Autodesk Inventor part; units mm, degrees
(part 3 of 3)
sketch "Эскиз17" plane through (0, 0, 0) normal (0, 0, -1) x (-1, 0, 0)
  arc A0 (-173.7802, -1.8121) -> (-173.9729, -1.8158) centre (-173.7802, -6.8121) ccw projected
  line L0 (-173.7802, -1.8121) -> (-160.0497, -1.8121) projected
  arc A1 (-152.9786, -18.8832) -> (-160.0497, -1.8121) centre (-160.0497, -11.8121) ccw projected
  line L1 (-152.9786, -18.8832) -> (-158.214, -24.1186) projected
  arc A2 (-164.3429, -27.0031) -> (-158.214, -24.1186) centre (-165.2851, -17.0475) ccw projected
  arc A3 (-173.9729, -1.8158) -> (-164.3429, -27.0031) centre (-132.2862, -0.3121) ccw projected
  line L2 (-174, 36.762) -> (-174, 1.1879) projected
  arc A4 (-171.0229, 35.5585) -> (-174, 36.762) centre (-174.2862, 31.7702) ccw projected
  arc A5 (-153.0118, 17.836) -> (-171.0229, 35.5585) centre (-295.6146, -109.0766) ccw projected
  arc A6 (-160.4818, 1.1879) -> (-153.0118, 17.836) centre (-160.4818, 11.1879) ccw projected
  line L3 (-160.4818, 1.1879) -> (-174, 1.1879) projected
  line L4 (-179, 51.6879) -> (181.2748, 51.6879) projected
  line L5 (-179, -0.3121) -> (-179, 51.6879) projected
  arc A7 (-179, -0.3121) -> (-165.3495, -33.3121) centre (-132.2862, -0.3121) ccw projected
  line L6 (-165.3495, -33.3121) -> (167.6243, -33.3121) projected
  arc A8 (167.6243, -33.3121) -> (181.2748, -0.3121) centre (134.5611, -0.3121) ccw projected
  line L7 (181.2748, 51.6879) -> (181.2748, -0.3121) projected
  line L8 (176.2748, 1.1879) -> (176.2748, 36.762) projected
  line L9 (176.2748, 1.1879) -> (162.7567, 1.1879) projected
  arc A9 (155.2866, 17.836) -> (162.7567, 1.1879) centre (162.7567, 11.1879) ccw projected
  arc A10 (173.2978, 35.5585) -> (155.2866, 17.836) centre (297.8894, -109.0766) ccw projected
  arc A11 (176.2748, 36.762) -> (173.2978, 35.5585) centre (176.5611, 31.7702) ccw projected
  arc A12 (-128.2552, 14.1361) -> (-136.3136, 14.1371) centre (-132.2862, -0.3121) ccw projected
  arc A13 (-145.382, 16.0725) -> (-136.3136, 14.1371) centre (-138.9985, 23.7699) ccw projected
  arc A14 (-168.1568, 38.4246) -> (-145.382, 16.0725) centre (-23.5217, 163.0162) ccw projected
  arc A15 (-164.3686, 46.6879) -> (-168.1568, 38.4246) centre (-164.3686, 41.6879) ccw projected
  line L10 (-164.3686, 46.6879) -> (-100.194, 46.6879) projected
  arc A16 (-96.4037, 38.427) -> (-100.194, 46.6879) centre (-100.194, 41.6879) ccw projected
  arc A17 (-119.19, 16.0661) -> (-96.4037, 38.427) centre (-240.0147, 161.9803) ccw projected
  arc A18 (-128.2552, 14.1361) -> (-119.19, 16.0661) centre (-125.5679, 23.7682) ccw projected
  arc A19 (170.4316, 38.4246) -> (166.6434, 46.6879) centre (166.6434, 41.6879) ccw projected
  arc A20 (147.6568, 16.0725) -> (170.4316, 38.4246) centre (25.7966, 163.0162) ccw projected
  arc A21 (138.5884, 14.1371) -> (147.6568, 16.0725) centre (141.2733, 23.7699) ccw projected
  arc A22 (138.5884, 14.1371) -> (130.53, 14.1361) centre (134.5611, -0.3121) ccw projected
  arc A23 (121.4649, 16.0661) -> (130.53, 14.1361) centre (127.8427, 23.7682) ccw projected
  arc A24 (98.6785, 38.427) -> (121.4649, 16.0661) centre (242.2895, 161.9803) ccw projected
  arc A25 (102.4688, 46.6879) -> (98.6785, 38.427) centre (102.4688, 41.6879) ccw projected
  line L11 (102.4688, 46.6879) -> (166.6434, 46.6879) projected
  arc A26 (77.8151, 38.3038) -> (74.1343, 46.6879) centre (74.1343, 41.6879) ccw projected
  line L12 (77.8151, 38.3038) -> (51.7107, 9.911) projected
  arc A27 (36.9877, 9.911) -> (51.7107, 9.911) centre (44.3492, 16.6792) ccw projected
  line L13 (36.9877, 9.911) -> (10.8834, 38.3038) projected
  arc A28 (14.5641, 46.6879) -> (10.8834, 38.3038) centre (14.5641, 41.6879) ccw projected
  line L14 (14.5641, 46.6879) -> (74.1343, 46.6879) projected
  line L15 (-49.4359, 9.911) -> (-75.5403, 38.3038) projected
  arc A29 (-71.8595, 46.6879) -> (-75.5403, 38.3038) centre (-71.8595, 41.6879) ccw projected
  line L16 (-71.8595, 46.6879) -> (-12.2893, 46.6879) projected
  arc A30 (-8.6085, 38.3038) -> (-12.2893, 46.6879) centre (-12.2893, 41.6879) ccw projected
  line L17 (-8.6085, 38.3038) -> (-34.7129, 9.911) projected
  arc A31 (-49.4359, 9.911) -> (-34.7129, 9.911) centre (-42.0744, 16.6792) ccw projected
  arc A32 (166.6178, -27.0031) -> (176.2477, -1.8158) centre (134.5611, -0.3121) ccw projected
  arc A33 (160.4889, -24.1186) -> (166.6178, -27.0031) centre (167.5599, -17.0475) ccw projected
  line L18 (160.4889, -24.1186) -> (155.2534, -18.8832) projected
  arc A34 (162.3245, -1.8121) -> (155.2534, -18.8832) centre (162.3245, -11.8121) ccw projected
  line L19 (162.3245, -1.8121) -> (176.055, -1.8121) projected
  arc A35 (176.2477, -1.8158) -> (176.055, -1.8121) centre (176.055, -6.8121) ccw projected
  circle A36 centre (-85.2862, 46.6879) radius 2.1 projected
  circle A37 centre (1.1374, 46.6879) radius 2.1 projected
  circle A38 centre (87.5611, 46.6879) radius 2.1 projected
  circle A39 centre (-123.2862, -0.3121) radius 2.1 projected
  circle A40 centre (-132.2862, 8.6879) radius 2.1 projected
  circle A41 centre (125.5611, -0.3121) radius 2.1 projected
  circle A42 centre (134.5611, -9.3121) radius 2.1 projected
  circle A43 centre (134.5611, 8.6879) radius 2.1 projected
  circle A44 centre (-132.2862, -0.3121) radius 4 projected
  circle A45 centre (-132.2862, -9.3121) radius 2.1 projected
  circle A46 centre (-141.2862, -0.3121) radius 2.1 projected
  circle A47 centre (143.5611, -0.3121) radius 2.1 projected
  circle A48 centre (134.5611, -0.3121) radius 4 projected
  line L20 (129.2891, -28.3121) -> (116.1593, -28.3121) projected
  arc A49 (114.1289, -23.1036) -> (116.1593, -28.3121) centre (116.1593, -25.3121) ccw projected
  arc A50 (116.4129, -21.0376) -> (114.1289, -23.1036) centre (243.3255, -163.6405) ccw projected
  arc A51 (131.9582, -23.9426) -> (116.4129, -21.0376) centre (123.0611, -28.5077) ccw projected
  arc A52 (129.2891, -28.3121) -> (131.9582, -23.9426) centre (129.2891, -25.3121) ccw projected
  line L21 (153.1971, -28.3121) -> (139.6296, -28.3121) projected
  arc A53 (136.8733, -24.1278) -> (139.6296, -28.3121) centre (139.6296, -25.3121) ccw projected
  arc A54 (153.1321, -21.0045) -> (136.8733, -24.1278) centre (146.0611, -28.0756) ccw projected
  line L22 (153.1321, -21.0045) -> (155.3184, -23.1908) projected
  arc A55 (153.1971, -28.3121) -> (155.3184, -23.1908) centre (153.1971, -25.3121) ccw projected
  line L23 (89.0611, -12.0997) -> (89.0611, 30.4755) projected
  arc A56 (97.3626, 34.2305) -> (89.0611, 30.4755) centre (94.0611, 30.4755) ccw projected
  arc A57 (118.1829, 12.7841) -> (97.3626, 34.2305) centre (-27.7313, -108.0406) ccw projected
  arc A58 (120.1128, 3.7189) -> (118.1829, 12.7841) centre (110.4807, 6.4063) ccw projected
  arc A59 (120.1128, 3.7189) -> (120.1118, -4.3395) centre (134.5611, -0.3121) ccw projected
  arc A60 (118.1765, -13.4079) -> (120.1118, -4.3395) centre (110.479, -7.0244) ccw projected
  arc A61 (105.2981, -27.4478) -> (118.1765, -13.4079) centre (-28.7673, 108.4524) ccw projected
  arc A62 (103.1912, -28.3121) -> (105.2981, -27.4478) centre (103.1912, -25.3121) ccw projected
  line L24 (103.1912, -28.3121) -> (102.4688, -28.3121) projected
  arc A63 (89.0611, -12.0997) -> (102.4688, -28.3121) centre (107.9833, -10.1012) ccw projected
  line L25 (-137.3548, -28.3121) -> (-150.9223, -28.3121) projected
  arc A64 (-153.0436, -23.1908) -> (-150.9223, -28.3121) centre (-150.9223, -25.3121) ccw projected
  line L26 (-153.0436, -23.1908) -> (-150.8573, -21.0045) projected
  arc A65 (-134.5985, -24.1278) -> (-150.8573, -21.0045) centre (-143.7862, -28.0756) ccw projected
  arc A66 (-137.3548, -28.3121) -> (-134.5985, -24.1278) centre (-137.3548, -25.3121) ccw projected
  line L27 (61.2667, -23.2817) -> (68.6995, -15.1972) projected
  arc A67 (86.0611, -21.9654) -> (68.6995, -15.1972) centre (76.0611, -21.9654) ccw projected
  arc A68 (74.9266, -28.3121) -> (86.0611, -21.9654) centre (74.5305, -14.6768) ccw projected
  line L28 (74.9266, -28.3121) -> (63.4752, -28.3121) projected
  arc A69 (61.2667, -23.2817) -> (63.4752, -28.3121) centre (63.4752, -25.3121) ccw projected
  arc A70 (70.312, 20.2554) -> (27.9585, -23.6784) centre (162.6046, -111.0994) ccw projected
  arc A71 (86.0611, 12.0731) -> (70.312, 20.2554) centre (76.0611, 12.0731) ccw projected
  line L29 (86.0611, 12.0731) -> (86.0611, 12.0172) projected
  arc A72 (83.4226, 5.249) -> (86.0611, 12.0172) centre (76.0611, 12.0172) ccw projected
  line L30 (83.4226, 5.249) -> (53.4579, -27.3426) projected
  arc A73 (51.2494, -28.3121) -> (53.4579, -27.3426) centre (51.2494, -25.3121) ccw projected
  line L31 (51.2494, -28.3121) -> (30.4747, -28.3121) projected
  arc A74 (27.9585, -23.6784) -> (30.4747, -28.3121) centre (30.4747, -25.3121) ccw projected
  line L32 (2.6374, -14.6768) -> (2.6374, 30.0143) projected
  arc A75 (11.3182, 33.3984) -> (2.6374, 30.0143) centre (7.6374, 30.0143) ccw projected
  line L33 (11.3182, 33.3984) -> (36.0889, 6.4561) projected
  arc A76 (36.0889, -7.0803) -> (36.0889, 6.4561) centre (28.7274, -0.3121) ccw projected
  line L34 (36.0889, -7.0803) -> (17.4598, -27.3426) projected
  arc A77 (15.2513, -28.3121) -> (17.4598, -27.3426) centre (15.2513, -25.3121) ccw projected
  line L35 (15.2513, -28.3121) -> (14.5641, -28.3121) projected
  arc A78 (2.6374, -14.6768) -> (14.5641, -28.3121) centre (18.1319, -13.1577) ccw projected
  line L36 (-113.8844, -28.3121) -> (-127.0142, -28.3121) projected
  arc A79 (-129.6834, -23.9426) -> (-127.0142, -28.3121) centre (-127.0142, -25.3121) ccw projected
  arc A80 (-114.1381, -21.0376) -> (-129.6834, -23.9426) centre (-120.7862, -28.5077) ccw projected
  arc A81 (-111.8541, -23.1036) -> (-114.1381, -21.0376) centre (-241.0507, -163.6405) ccw projected
  arc A82 (-113.8844, -28.3121) -> (-111.8541, -23.1036) centre (-113.8844, -25.3121) ccw projected
  line L37 (-15.185, -27.3426) -> (-33.8141, -7.0803) projected
  arc A83 (-33.8141, 6.4561) -> (-33.8141, -7.0803) centre (-26.4526, -0.3121) ccw projected
  line L38 (-33.8141, 6.4561) -> (-9.0433, 33.3984) projected
  arc A84 (-0.3626, 30.0143) -> (-9.0433, 33.3984) centre (-5.3626, 30.0143) ccw projected
  line L39 (-0.3626, 30.0143) -> (-0.3626, -14.6768) projected
  arc A85 (-12.2893, -28.3121) -> (-0.3626, -14.6768) centre (-15.857, -13.1577) ccw projected
  line L40 (-12.2893, -28.3121) -> (-12.9765, -28.3121) projected
  arc A86 (-15.185, -27.3426) -> (-12.9765, -28.3121) centre (-12.9765, -25.3121) ccw projected
  line L41 (-51.183, -27.3426) -> (-81.1477, 5.249) projected
  arc A87 (-83.7862, 12.0172) -> (-81.1477, 5.249) centre (-73.7862, 12.0172) ccw projected
  line L42 (-83.7862, 12.0172) -> (-83.7862, 12.0731) projected
  arc A88 (-68.0372, 20.2554) -> (-83.7862, 12.0731) centre (-73.7862, 12.0731) ccw projected
  arc A89 (-25.6837, -23.6784) -> (-68.0372, 20.2554) centre (-160.3298, -111.0994) ccw projected
  arc A90 (-28.1999, -28.3121) -> (-25.6837, -23.6784) centre (-28.1999, -25.3121) ccw projected
  line L43 (-28.1999, -28.3121) -> (-48.9746, -28.3121) projected
  arc A91 (-51.183, -27.3426) -> (-48.9746, -28.3121) centre (-48.9746, -25.3121) ccw projected
  line L44 (-100.194, -28.3121) -> (-100.9164, -28.3121) projected
  arc A92 (-103.0232, -27.4478) -> (-100.9164, -28.3121) centre (-100.9164, -25.3121) ccw projected
  arc A93 (-115.9016, -13.4079) -> (-103.0232, -27.4478) centre (31.0421, 108.4524) ccw projected
  arc A94 (-117.837, -4.3395) -> (-115.9016, -13.4079) centre (-108.2042, -7.0244) ccw projected
  arc A95 (-117.837, -4.3395) -> (-117.838, 3.7189) centre (-132.2862, -0.3121) ccw projected
  arc A96 (-115.908, 12.7841) -> (-117.838, 3.7189) centre (-108.2059, 6.4063) ccw projected
  arc A97 (-95.0878, 34.2305) -> (-115.908, 12.7841) centre (30.0061, -108.0406) ccw projected
  arc A98 (-86.7862, 30.4755) -> (-95.0878, 34.2305) centre (-91.7862, 30.4755) ccw projected
  line L45 (-86.7862, 30.4755) -> (-86.7862, -12.0997) projected
  arc A99 (-100.194, -28.3121) -> (-86.7862, -12.0997) centre (-105.7085, -10.1012) ccw projected
  arc A100 (-66.4247, -15.1972) -> (-83.7862, -21.9654) centre (-73.7862, -21.9654) ccw projected
  line L46 (-66.4247, -15.1972) -> (-58.9919, -23.2817) projected
  arc A101 (-61.2003, -28.3121) -> (-58.9919, -23.2817) centre (-61.2003, -25.3121) ccw projected
  line L47 (-61.2003, -28.3121) -> (-72.6518, -28.3121) projected
  arc A102 (-83.7862, -21.9654) -> (-72.6518, -28.3121) centre (-72.2556, -14.6768) ccw projected
  circle A103 centre (87.5611, -28.3121) radius 2.1 projected
  circle A104 centre (1.1374, -28.3121) radius 2.1 projected
  circle A105 centre (-85.2862, -28.3121) radius 2.1 projected
  line L48 (1.1374, -33.3121) -> (1.1374, -21.3121)
  line L49 (1.1374, -21.3121) -> (-186, -21.3121)
  line L50 (1.1374, -21.3121) -> (188.2748, -21.3121)
  point P0 (0, 0)
  point P1 (176.2885, -21.3121)
  point P2 (170.6032, -21.3121)
  point P3 (157.6824, -21.3121)
  point P4 (153.4397, -21.3121)
  point P5 (138.6952, -21.3121)
  point P6 (130.0053, -21.3121)
  point P7 (116.1052, -21.3121)
  point P8 (111.2454, -21.3121)
  point P9 (92.6092, -21.3121)
  point P10 (86.0397, -21.3121)
  point P11 (63.0775, -21.3121)
  point P12 (59.0023, -21.3121)
  point P13 (29.5248, -21.3121)
  point P14 (23.0042, -21.3121)
  point P15 (4.8695, -21.3121)
  point P16 (-2.5946, -21.3121)
  point P17 (-20.7294, -21.3121)
  point P18 (-27.25, -21.3121)
  point P19 (-56.7274, -21.3121)
  point P20 (-60.8027, -21.3121)
  point P21 (-83.7649, -21.3121)
  point P22 (-90.3344, -21.3121)
  point P23 (-108.9706, -21.3121)
  point P24 (-113.8303, -21.3121)
  point P25 (-127.7305, -21.3121)
  point P26 (-136.4204, -21.3121)
  point P27 (-151.1649, -21.3121)
  point P28 (-155.4075, -21.3121)
  point P29 (-168.3284, -21.3121)
  point P30 (-174.0136, -21.3121)
  dimension "d128" = 12
  constraints: 6 end point, 1 midpoint, 1 perpendicular, 1 symmetric about line, 1 vertical
  measures "d128" distance of L48.start L48.end
extrude "Выдавливание13" cut sketch "Эскиз17" against normal blind 10 contours A3 A2 L1 L49 L26 A64 L25 A66 A65 A80 A79 L36 A82 A81 A93 A92 L44 A99 A100 A102 L47 A101 L46 L41 A91 L43 A90 A89 L37 A86 L40 A85 L48 A104 L6 A7 | L48 A104 L50 A78 L35 A77 L34 A70 A74 L31 A73 L30 L27 A69 L28 A68 A67 A63 L24 A62 A61 A50 A49 L20 A52 A51 A54 A53 L21 A55 L22 L18 A33 A32 A8 L6
sketch "Эскиз18" plane through (0, 0, 0) normal (0, 0, -1) x (-1, 0, 0)
  circle A0 centre (134.5611, -0.3121) radius 4 projected
  circle A1 centre (143.5611, -0.3121) radius 2.1 projected
  circle A2 centre (-141.2862, -0.3121) radius 2.1 projected
  circle A3 centre (-132.2862, -9.3121) radius 2.1 projected
  circle A4 centre (-132.2862, -0.3121) radius 4 projected
  circle A5 centre (134.5611, 8.6879) radius 2.1 projected
  circle A6 centre (134.5611, -9.3121) radius 2.1 projected
  circle A7 centre (125.5611, -0.3121) radius 2.1 projected
  circle A8 centre (-132.2862, 8.6879) radius 2.1 projected
  circle A9 centre (-123.2862, -0.3121) radius 2.1 projected
  circle A10 centre (87.5611, 46.6879) radius 2.1 projected
  circle A11 centre (1.1374, 46.6879) radius 2.1 projected
  circle A12 centre (-85.2862, 46.6879) radius 2.1 projected
  line L0 (-49.4359, 9.911) -> (-75.5403, 38.3038) projected
  arc A13 (-71.8595, 46.6879) -> (-75.5403, 38.3038) centre (-71.8595, 41.6879) ccw projected
  line L1 (-71.8595, 46.6879) -> (-12.2893, 46.6879) projected
  arc A14 (-8.6085, 38.3038) -> (-12.2893, 46.6879) centre (-12.2893, 41.6879) ccw projected
  line L2 (-8.6085, 38.3038) -> (-34.7129, 9.911) projected
  arc A15 (-49.4359, 9.911) -> (-34.7129, 9.911) centre (-42.0744, 16.6792) ccw projected
  arc A16 (77.8151, 38.3038) -> (74.1343, 46.6879) centre (74.1343, 41.6879) ccw projected
  line L3 (77.8151, 38.3038) -> (51.7107, 9.911) projected
  arc A17 (36.9877, 9.911) -> (51.7107, 9.911) centre (44.3492, 16.6792) ccw projected
  line L4 (36.9877, 9.911) -> (10.8834, 38.3038) projected
  arc A18 (14.5641, 46.6879) -> (10.8834, 38.3038) centre (14.5641, 41.6879) ccw projected
  line L5 (14.5641, 46.6879) -> (74.1343, 46.6879) projected
  arc A19 (170.4316, 38.4246) -> (166.6434, 46.6879) centre (166.6434, 41.6879) ccw projected
  arc A20 (147.6568, 16.0725) -> (170.4316, 38.4246) centre (25.7966, 163.0162) ccw projected
  arc A21 (138.5884, 14.1371) -> (147.6568, 16.0725) centre (141.2733, 23.7699) ccw projected
  arc A22 (138.5884, 14.1371) -> (130.53, 14.1361) centre (134.5611, -0.3121) ccw projected
  arc A23 (121.4649, 16.0661) -> (130.53, 14.1361) centre (127.8427, 23.7682) ccw projected
  arc A24 (98.6785, 38.427) -> (121.4649, 16.0661) centre (242.2895, 161.9803) ccw projected
  arc A25 (102.4688, 46.6879) -> (98.6785, 38.427) centre (102.4688, 41.6879) ccw projected
  line L6 (102.4688, 46.6879) -> (166.6434, 46.6879) projected
  arc A26 (-128.2552, 14.1361) -> (-136.3136, 14.1371) centre (-132.2862, -0.3121) ccw projected
  arc A27 (-145.382, 16.0725) -> (-136.3136, 14.1371) centre (-138.9985, 23.7699) ccw projected
  arc A28 (-168.1568, 38.4246) -> (-145.382, 16.0725) centre (-23.5217, 163.0162) ccw projected
  arc A29 (-164.3686, 46.6879) -> (-168.1568, 38.4246) centre (-164.3686, 41.6879) ccw projected
  line L7 (-164.3686, 46.6879) -> (-100.194, 46.6879) projected
  arc A30 (-96.4037, 38.427) -> (-100.194, 46.6879) centre (-100.194, 41.6879) ccw projected
  arc A31 (-119.19, 16.0661) -> (-96.4037, 38.427) centre (-240.0147, 161.9803) ccw projected
  arc A32 (-128.2552, 14.1361) -> (-119.19, 16.0661) centre (-125.5679, 23.7682) ccw projected
  line L8 (176.2748, 1.1879) -> (176.2748, 36.762) projected
  line L9 (176.2748, 1.1879) -> (162.7567, 1.1879) projected
  arc A33 (155.2866, 17.836) -> (162.7567, 1.1879) centre (162.7567, 11.1879) ccw projected
  arc A34 (173.2978, 35.5585) -> (155.2866, 17.836) centre (297.8894, -109.0766) ccw projected
  arc A35 (176.2748, 36.762) -> (173.2978, 35.5585) centre (176.5611, 31.7702) ccw projected
  line L10 (-2.5946, -21.3121) -> (4.8695, -21.3121) projected
  arc A36 (2.6374, -14.6768) -> (4.8695, -21.3121) centre (18.1319, -13.1577) ccw projected
  line L11 (2.6374, -14.6768) -> (2.6374, 30.0143) projected
  arc A37 (11.3182, 33.3984) -> (2.6374, 30.0143) centre (7.6374, 30.0143) ccw projected
  line L12 (11.3182, 33.3984) -> (36.0889, 6.4561) projected
  arc A38 (36.0889, -7.0803) -> (36.0889, 6.4561) centre (28.7274, -0.3121) ccw projected
  line L13 (36.0889, -7.0803) -> (23.0042, -21.3121) projected
  line L14 (23.0042, -21.3121) -> (29.5248, -21.3121) projected
  arc A39 (70.312, 20.2554) -> (29.5248, -21.3121) centre (162.6046, -111.0994) ccw projected
  arc A40 (86.0611, 12.0731) -> (70.312, 20.2554) centre (76.0611, 12.0731) ccw projected
  line L15 (86.0611, 12.0731) -> (86.0611, 12.0172) projected
  arc A41 (83.4226, 5.249) -> (86.0611, 12.0172) centre (76.0611, 12.0172) ccw projected
  line L16 (83.4226, 5.249) -> (59.0023, -21.3121) projected
  line L17 (59.0023, -21.3121) -> (63.0775, -21.3121) projected
  line L18 (63.0775, -21.3121) -> (68.6995, -15.1972) projected
  arc A42 (86.0397, -21.3121) -> (68.6995, -15.1972) centre (76.0611, -21.9654) ccw projected
  line L19 (86.0397, -21.3121) -> (92.6092, -21.3121) projected
  arc A43 (89.0611, -12.0997) -> (92.6092, -21.3121) centre (107.9833, -10.1012) ccw projected
  line L20 (89.0611, -12.0997) -> (89.0611, 30.4755) projected
  arc A44 (97.3626, 34.2305) -> (89.0611, 30.4755) centre (94.0611, 30.4755) ccw projected
  arc A45 (118.1829, 12.7841) -> (97.3626, 34.2305) centre (-27.7313, -108.0406) ccw projected
  arc A46 (120.1128, 3.7189) -> (118.1829, 12.7841) centre (110.4807, 6.4063) ccw projected
  arc A47 (120.1128, 3.7189) -> (120.1118, -4.3395) centre (134.5611, -0.3121) ccw projected
  arc A48 (118.1765, -13.4079) -> (120.1118, -4.3395) centre (110.479, -7.0244) ccw projected
  arc A49 (111.2454, -21.3121) -> (118.1765, -13.4079) centre (-28.7673, 108.4524) ccw projected
  line L21 (111.2454, -21.3121) -> (116.1052, -21.3121) projected
  arc A50 (116.4129, -21.0376) -> (116.1052, -21.3121) centre (243.3255, -163.6405) ccw projected
  arc A51 (130.0053, -21.3121) -> (116.4129, -21.0376) centre (123.0611, -28.5077) ccw projected
  line L22 (130.0053, -21.3121) -> (138.6952, -21.3121) projected
  arc A52 (153.1321, -21.0045) -> (138.6952, -21.3121) centre (146.0611, -28.0756) ccw projected
  line L23 (153.1321, -21.0045) -> (153.4397, -21.3121) projected
  line L24 (153.4397, -21.3121) -> (157.6824, -21.3121) projected
  line L25 (157.6824, -21.3121) -> (155.2534, -18.8832) projected
  arc A53 (162.3245, -1.8121) -> (155.2534, -18.8832) centre (162.3245, -11.8121) ccw projected
  line L26 (162.3245, -1.8121) -> (176.055, -1.8121) projected
  arc A54 (176.2477, -1.8158) -> (176.055, -1.8121) centre (176.055, -6.8121) ccw projected
  arc A55 (170.6032, -21.3121) -> (176.2477, -1.8158) centre (134.5611, -0.3121) ccw projected
  line L27 (170.6032, -21.3121) -> (176.2885, -21.3121) projected
  arc A56 (176.2885, -21.3121) -> (181.2748, -0.3121) centre (134.5611, -0.3121) ccw projected
  line L28 (181.2748, 51.6879) -> (181.2748, -0.3121) projected
  line L29 (-179, 51.6879) -> (181.2748, 51.6879) projected
  line L30 (-179, -0.3121) -> (-179, 51.6879) projected
  arc A57 (-179, -0.3121) -> (-174.0136, -21.3121) centre (-132.2862, -0.3121) ccw projected
  line L31 (-174.0136, -21.3121) -> (-168.3284, -21.3121) projected
  arc A58 (-173.9729, -1.8158) -> (-168.3284, -21.3121) centre (-132.2862, -0.3121) ccw projected
  arc A59 (-173.7802, -1.8121) -> (-173.9729, -1.8158) centre (-173.7802, -6.8121) ccw projected
  line L32 (-173.7802, -1.8121) -> (-160.0497, -1.8121) projected
  arc A60 (-152.9786, -18.8832) -> (-160.0497, -1.8121) centre (-160.0497, -11.8121) ccw projected
  line L33 (-152.9786, -18.8832) -> (-155.4075, -21.3121) projected
  line L34 (-155.4075, -21.3121) -> (-151.1649, -21.3121) projected
  line L35 (-151.1649, -21.3121) -> (-150.8573, -21.0045) projected
  arc A61 (-136.4204, -21.3121) -> (-150.8573, -21.0045) centre (-143.7862, -28.0756) ccw projected
  line L36 (-136.4204, -21.3121) -> (-127.7305, -21.3121) projected
  arc A62 (-114.1381, -21.0376) -> (-127.7305, -21.3121) centre (-120.7862, -28.5077) ccw projected
  arc A63 (-113.8303, -21.3121) -> (-114.1381, -21.0376) centre (-241.0507, -163.6405) ccw projected
  line L37 (-113.8303, -21.3121) -> (-108.9706, -21.3121) projected
  arc A64 (-115.9016, -13.4079) -> (-108.9706, -21.3121) centre (31.0421, 108.4524) ccw projected
  arc A65 (-117.837, -4.3395) -> (-115.9016, -13.4079) centre (-108.2042, -7.0244) ccw projected
  arc A66 (-117.837, -4.3395) -> (-117.838, 3.7189) centre (-132.2862, -0.3121) ccw projected
  arc A67 (-115.908, 12.7841) -> (-117.838, 3.7189) centre (-108.2059, 6.4063) ccw projected
  arc A68 (-95.0878, 34.2305) -> (-115.908, 12.7841) centre (30.0061, -108.0406) ccw projected
  arc A69 (-86.7862, 30.4755) -> (-95.0878, 34.2305) centre (-91.7862, 30.4755) ccw projected
  line L38 (-86.7862, 30.4755) -> (-86.7862, -12.0997) projected
  arc A70 (-90.3344, -21.3121) -> (-86.7862, -12.0997) centre (-105.7085, -10.1012) ccw projected
  line L39 (-90.3344, -21.3121) -> (-83.7649, -21.3121) projected
  arc A71 (-66.4247, -15.1972) -> (-83.7649, -21.3121) centre (-73.7862, -21.9654) ccw projected
  line L40 (-66.4247, -15.1972) -> (-60.8027, -21.3121) projected
  line L41 (-60.8027, -21.3121) -> (-56.7274, -21.3121) projected
  line L42 (-56.7274, -21.3121) -> (-81.1477, 5.249) projected
  arc A72 (-83.7862, 12.0172) -> (-81.1477, 5.249) centre (-73.7862, 12.0172) ccw projected
  line L43 (-83.7862, 12.0172) -> (-83.7862, 12.0731) projected
  arc A73 (-68.0372, 20.2554) -> (-83.7862, 12.0731) centre (-73.7862, 12.0731) ccw projected
  arc A74 (-27.25, -21.3121) -> (-68.0372, 20.2554) centre (-160.3298, -111.0994) ccw projected
  line L44 (-27.25, -21.3121) -> (-20.7294, -21.3121) projected
  line L45 (-20.7294, -21.3121) -> (-33.8141, -7.0803) projected
  arc A75 (-33.8141, 6.4561) -> (-33.8141, -7.0803) centre (-26.4526, -0.3121) ccw projected
  line L46 (-33.8141, 6.4561) -> (-9.0433, 33.3984) projected
  arc A76 (-0.3626, 30.0143) -> (-9.0433, 33.3984) centre (-5.3626, 30.0143) ccw projected
  line L47 (-0.3626, 30.0143) -> (-0.3626, -14.6768) projected
  arc A77 (-2.5946, -21.3121) -> (-0.3626, -14.6768) centre (-15.857, -13.1577) ccw projected
  line L48 (-174, 36.762) -> (-174, 1.1879) projected
  arc A78 (-171.0229, 35.5585) -> (-174, 36.762) centre (-174.2862, 31.7702) ccw projected
  arc A79 (-153.0118, 17.836) -> (-171.0229, 35.5585) centre (-295.6146, -109.0766) ccw projected
  arc A80 (-160.4818, 1.1879) -> (-153.0118, 17.836) centre (-160.4818, 11.1879) ccw projected
  line L49 (-160.4818, 1.1879) -> (-174, 1.1879) projected
  line L50 (1.1374, 51.6879) -> (1.1374, -14.2121)
  line L51 (1.1374, 15.1879) -> (-9.5938, 15.1879)
  circle A81 centre (87.5611, -16.3121) radius 2.1
  circle A82 centre (1.1374, -16.3121) radius 2.1
  circle A83 centre (-85.2862, -16.3121) radius 2.1
  arc A84 (2.6374, -14.6768) -> (23.0042, -21.3121) centre (14.0337, -14.2715) ccw
  arc A85 (-108.9706, -21.3121) -> (-90.3344, -21.3121) centre (-99.6525, -12.6761) ccw
  line L52 (1.1374, -21.3121) -> (176.2885, -21.3121)
  line L53 (1.1374, -16.3121) -> (1.1374, -18.4121)
  line L54 (1.1374, -21.3121) -> (-174.0136, -21.3121)
  line L55 (-179, 51.6879) -> (181.2748, 51.6879)
  line L56 (181.2748, 51.6879) -> (181.2748, 56.6879)
  line L57 (181.2748, 56.6879) -> (-179, 56.6879)
  line L58 (-179, 56.6879) -> (-179, 51.6879)
  line L59 (-176.1745, -16.3121) -> (-87.3862, -16.3121)
  line L60 (-83.1862, -16.3121) -> (-0.6112, -16.3121)
  line L61 (178.4493, -16.3121) -> (89.6611, -16.3121)
  line L62 (85.4611, -16.3121) -> (2.8143, -16.3121)
  line L63 (-174, 36.762) -> (-174, 68)
  circle A86 centre (-174, 51.6879) radius 2.1
  circle A87 centre (176.2748, 51.6879) radius 2.1
  point P0 (0, 0)
  dimension "d132" = 5
  dimension "d133" = 4.2
  constraints: 28 end point, 16 point on circle, 7 centre point, 6 parallel, 4 horizontal, 4 symmetric about line, 3 point on line, 2 midpoint, 1 perpendicular, 1 tangent, 1 vertical, 4 other
  measures "d132" distance of L55.end L56.end
  measures "d133" diameter of A86
